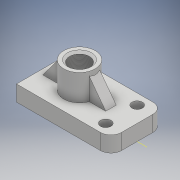
# Autodesk Inventor part: Деталь1
Saved by Autodesk Inventor 2018 (Build 220112000, 112)
## iProperties
Created: 2020-04-14
Part Number: Деталь1
Material: Типовые
Document SubType Name: Modeling
Designer: 2000
Density: 1 g/cm^3
Appearance: По умолчанию
Mass: 73.9169 g
Surface Area: 181.793 cm^2
Volume: 73.9169 cm^3
Author: 2000
Autodesk Inventor part; units mm, degrees
ref_plane "YZ Plane" through (0, 0, 0) normal (1, 0, 0) x (0, 1, 0)
ref_plane "XZ Plane" through (0, 0, 0) normal (0, 1, 0) x (-1, 0, 0)
ref_plane "XY Plane" through (0, 0, 0) normal (0, 0, 1) x (1, 0, 0)
sketch "Эскиз1" plane through (0, 0, 0) normal (0, 0, 1) x (1, 0, 0)
  line L0 (-35, 25) -> (45, 25)
  line L1 (55, 15) -> (55, -15)
  line L2 (45, -25) -> (-35, -25)
  line L3 (-35, -25) -> (-35, 25)
  arc A0 (55, 15) -> (45, 25) centre (45, 15) ccw
  arc A1 (45, -25) -> (55, -15) centre (45, -15) ccw
  point P0 (0, 0)
  point P1 (55, 25)
  dimension "d1" = 50
  dimension "d2" = 35
  dimension "d3" = 25
  dimension "d4" = 10
  dimension "d6" = 80
  constraints: 8 end point, 4 point on circle, 4 tangent, 2 centre point, 2 parallel, 2 point on line, 1 equal radius, 1 horizontal, 1 perpendicular
  measures "d1" distance of L2.end L0.start
  measures "d2" distance from line of L3 point (0, 0)
  measures "d3" distance from line of L0 point (0, 0)
  measures "d4" radius of A0
  measures "d6" distance of L0.start L0.end
extrude "Выдавливание1" add sketch "Эскиз1" along normal blind 15
sketch "Эскиз5" plane through (0, 0, 15) normal (0, 0, 1) x (1, 0, 0)
  circle A0 centre (0, 0) radius 15
  dimension "d32" = 30
  constraints: 1 centre point, 1 coincident
  measures "d32" diameter of A0
extrude "Выдавливание3" add sketch "Эскиз5" along normal blind 25
sketch "Эскиз6" plane through (0, 0, 40) normal (0, 0, 1) x (1, 0, 0)
  point P0 (0, 0)
hole "Отверстие3" at (0, 0, 40) direction (0, 0, -1) diameter 18.917 depth 45.1 thread size "M20x1" class "6H" standard "ISO Metric profile"
chamfer "Фаска2" distance 2 angle 45 1 edges at (0, 9.4585, 40)
sketch "Эскиз7" plane through (0, 0, 0) normal (0, 1, 0) x (-1, 0, 0)
  line L0 (-15, 35) -> (-30, 15)
  line L1 (-15, 15) -> (-15, 40) projected
  point P0 (0, 0)
  dimension "d45" = 5
  dimension "d46" = 15
  constraints: 2 end point, 1 horizontal alignment, 1 point on line
  measures "d45" distance of L1.end L0.start
  measures "d46" distance from line of L1 L0.end
extrude "Ребро жесткости1" add sketch "Эскиз7" along normal mid plane 10 rib yes fills toward (-22.46, 24.97) open curves L0
sketch "Эскиз8" plane through (0, 0, 0) normal (0, 1, 0) x (-1, 0, 0)
  line L0 (15, 35) -> (30, 15)
  line L1 (15, 15) -> (15, 40) projected
  line L2 (-14.1421, 15) -> (15, 15) projected
  point P0 (0, 0)
  point P1 (0.4289, 15)
  dimension "d53" = 5
  dimension "d54" = 15
  constraints: 2 end point, 1 horizontal alignment, 1 midpoint, 1 point on line
  measures "d53" distance of L1.end L0.start
  measures "d54" distance of L1.start L0.end
extrude "Ребро жесткости2" add sketch "Эскиз8" along normal mid plane 10 rib yes fills toward (22.46, 24.97) open curves L0
sketch "Эскиз9" plane through (0, 0, 15) normal (0, 0, 1) x (1, 0, 0)
  line L0 (-53, 0) -> (73, 0) projected
  point P0 (0, 0)
  point P1 (40, -15)
  point P2 (40, 15)
  dimension "d61" = 30
  dimension "d62" = 40
  constraints: 1 symmetric about line
  measures "d61" distance of point (40, 15) point (40, -15)
  measures "d62" horizontal distance of point (0, 0) point (40, 15)
hole "Отверстие4" at (40, -15, 15) at (40, 15, 15) direction (0, 0, -1) diameter 10 depth 15.1
